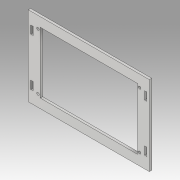
# Autodesk Inventor part: top_instrumentboard
Saved by Autodesk Inventor 2019.3 (Build 233278000, 278)
## iProperties
Created: 2019-05-28
Part Number: top_instrumentboard
Material: Generic
Document SubType Name: Modeling
Designer: Dave
Density: 1 g/cm^3
Appearance: Default
Author: Dave
Autodesk Inventor part; units mm, degrees
ref_plane "YZ Plane" through (0, 0, 0) normal (1, 0, 0) x (0, 1, 0)
ref_plane "XZ Plane" through (0, 0, 0) normal (0, 1, 0) x (-1, 0, 0)
ref_plane "XY Plane" through (0, 0, 0) normal (0, 0, 1) x (1, 0, 0)
sketch "Sketch1" plane through (0, 0, 0) normal (0, 0, 1) x (1, 0, 0)
  line L0 (0, 0) -> (152, 0)
  line L1 (152, 0) -> (152, 100)
  line L2 (152, 100) -> (0, 100)
  line L3 (0, 100) -> (0, 0)
  line L4 (15, 88.5) -> (137, 88.5)
  line L5 (137, 88.5) -> (137, 11.5)
  line L6 (137, 11.5) -> (15, 11.5)
  line L7 (15, 11.5) -> (15, 88.5)
  circle A0 centre (12.2, 85.3) radius 1.55
  circle A1 centre (12.2, 14.7) radius 1.55
  circle A2 centre (139.8, 85.3) radius 1.55
  circle A3 centre (139.8, 14.7) radius 1.55
  line L8 (0, 75) -> (0, 85)
  line L9 (0, 15) -> (0, 25)
  line L10 (152, 75) -> (152, 85)
  line L11 (152, 15) -> (152, 25)
  line L12 (3, 85) -> (6, 85)
  line L13 (6, 85) -> (6, 75)
  line L14 (6, 75) -> (3, 75)
  line L15 (3, 75) -> (3, 85)
  line L16 (3, 25) -> (6, 25)
  line L17 (6, 25) -> (6, 15)
  line L18 (6, 15) -> (3, 15)
  line L19 (3, 15) -> (3, 25)
  line L20 (149, 85) -> (146, 85)
  line L21 (146, 85) -> (146, 75)
  line L22 (146, 75) -> (149, 75)
  line L23 (149, 75) -> (149, 85)
  line L24 (149, 25) -> (146, 25)
  line L25 (146, 25) -> (146, 15)
  line L26 (146, 15) -> (149, 15)
  line L27 (149, 15) -> (149, 25)
  point P0 (76, 88.5)
  dimension "d0" = 122
  dimension "d1" = 77
  dimension "d3" = 15
  dimension "d5" = 11.5
  dimension "d6" = 3.1
  dimension "d7" = 127.6
  dimension "d8" = 63.8
  dimension "d9" = 70.6
  dimension "d10" = 3.2
  dimension "d11" = 3.2
  dimension "d14" = 100
  dimension "d15" = 11.5
  dimension "d16" = 152
  dimension "d17" = 15
  dimension "d22" = 3
  dimension "d23" = 10
  dimension "d24" = 3
  dimension "d25" = 3
  dimension "d26" = 15
  dimension "d27" = 15
  constraints: 56 end point, 12 parallel, 12 point on line, 6 horizontal, 6 perpendicular, 4 centre point, 3 equal radius, 2 collinear, 2 horizontal alignment, 2 vertical alignment, 1 midpoint
  measures "d0" distance of L4.start L4.end
  measures "d1" distance of L4.end L5.end
  measures "d3" distance between parallel lines of L1 L5
  measures "d5" distance between parallel lines of L6 L0
  measures "d6" diameter of A0
  measures "d7" distance of A2.centre A0.centre
  measures "d8" horizontal distance of A0.centre point (76, 88.5)
  measures "d9" distance of A3.centre A2.centre
  measures "d10" distance from line of L4 A0.centre
  measures "d11" distance from line of L6 A1.centre
  measures "d14" distance between parallel lines of L0 L2
  measures "d15" distance between parallel lines of L2 L4
  measures "d16" distance of L1.end L2.end
  measures "d17" distance between parallel lines of L3 L7
  measures "d22" distance of L12.start L12.end
  measures "d23" distance of L14.end L12.start
  measures "d24" distance between parallel lines of L3 L15
  measures "d25" distance between parallel lines of L1 L23
  measures "d26" distance between parallel lines of L0 L18
  measures "d27" distance between parallel lines of L2 L12
extrude "Extrusion1" add sketch "Sketch1" along normal blind 3
body "Solid1"
